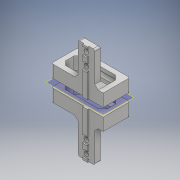
# Autodesk Inventor part: Estrutura - Suporte Mesa
Saved by Autodesk Inventor 2017 (Build 210142000, 142)
## iProperties
Created: 2020-08-23
Part Number: Estrutura - Suporte Mesa
Material: Generic
Document SubType Name: Modeling
Designer: ale
Density: 1 g/cm^3
Appearance: Default
Author: ale
Autodesk Inventor part; units mm, degrees
ref_plane "YZ Plane" through (0, 0, 0) normal (1, 0, 0) x (0, 1, 0)
ref_plane "XZ Plane" through (0, 0, 0) normal (0, 1, 0) x (-1, 0, 0)
ref_plane "XY Plane" through (0, 0, 0) normal (0, 0, 1) x (1, 0, 0)
sketch "Sketch1" plane through (0, 0, 0) normal (0, 0, 1) x (1, 0, 0)
  line L0 (-12.2491, 0) -> (12.2491, 0)
  line L1 (0, 10.917) -> (0, -10.917)
  line L2 (-40, -10) -> (-40, -16)
  line L3 (-40, -16) -> (16, -16)
  line L4 (-40, -10) -> (10, -10)
  line L5 (10, -10) -> (10, 10)
  line L6 (10, 10) -> (-40, 10)
  line L7 (-40, 10) -> (-40, 16)
  line L8 (-40, 16) -> (16, 16)
  line L9 (16, 16) -> (16, -16)
  point P0 (0, 0)
  point P1 (0, 0)
  dimension "d0" = 10
  dimension "d1" = 10
  dimension "d2" = 10
  dimension "d3" = 40
  dimension "d4" = 6
  dimension "d5" = 6
  dimension "d6" = 50
  dimension "d7" = 6
  constraints: 20 end point, 6 perpendicular, 2 horizontal, 2 midpoint, 2 vertical, 1 coincident
  measures "d0" distance between parallel lines of L6 L0
  measures "d1" distance between parallel lines of L4 L0
  measures "d2" distance between parallel lines of L5 L1
  measures "d3" distance between parallel lines of L2 L1
  measures "d4" distance between parallel lines of L3 L4
  measures "d5" distance between parallel lines of L9 L5
  measures "d6" distance between parallel lines of L7 L5
  measures "d7" distance between parallel lines of L6 L8
extrude "Extrusion1" add sketch "Sketch1" along normal blind 15 contours L5 L6 L7 L8 L9 L3 L2 L4
sketch "Sketch4" plane through (-40, 16, 0) normal (0, 1, 0) x (1, 0, 0)
  arc A0 (6, -4.25) -> (6, -10.75) centre (6, -7.5) ccw
  line L0 (0, 0) -> (0, -15) projected
  line L1 (56, 0) -> (0, 0) projected
  arc A1 (46, -10.75) -> (46, -4.25) centre (46, -7.5) ccw
  line L2 (56, -15) -> (0, -15) projected
  line L3 (46, -4.25) -> (6, -4.25)
  line L4 (46, -10.75) -> (6, -10.75)
  point P0 (40, 0)
  dimension "d22" = 6.5
  dimension "d23" = 6
  dimension "d24" = 7.5
  dimension "d25" = 6.5
  dimension "d26" = 46
  dimension "d27" = 7.5
  constraints: 4 end point, 4 point on circle, 4 tangent, 2 centre point
  measures "d22" diameter of A0
  measures "d23" distance from line of L0 A0.centre
  measures "d24" distance from line of L1 A0.centre
  measures "d25" diameter of A1
  measures "d26" distance from line of L0 A1.centre
  measures "d27" distance from line of L2 A1.centre
extrude "Extrusion3" cut sketch "Sketch4" against normal up to surface (6 mm away)
sketch "Sketch5" plane through (-40, -16, 0) normal (-1, 0, 0) x (0, 0, 1)
  line L0 (0, 0) -> (0, 32) projected
  line L1 (15, 6) -> (15, 0) projected
  line L2 (0, 32) -> (15, 32)
  line L3 (15, 32) -> (15, 0)
  line L4 (15, 0) -> (0, 0)
  line L5 (0, 0) -> (0, 32)
  point P0 (0, 16)
  constraints: 8 end point, 2 parallel, 1 horizontal, 1 perpendicular
extrude "Extrusion4" add sketch "Sketch5" along normal blind 6
sketch "Sketch6" plane through (16, -16, 0) normal (0, -1, 0) x (1, 0, 0)
  line L0 (-10, 0) -> (-30, 0)
  line L1 (-30, 0) -> (-30, 55)
  line L2 (-30, 55) -> (-10, 55)
  line L3 (-10, 55) -> (-10, 0)
  line L4 (-62, 0) -> (-62, 15) projected
  line L5 (0, 15) -> (-62, 15) projected
  point P0 (-16, 0)
  dimension "d43" = 20
  dimension "d44" = 55
  dimension "d76" = 52
  dimension "d77" = 15
  constraints: 8 end point, 2 parallel, 1 horizontal, 1 perpendicular
  measures "d43" distance of L1.end L2.end
  measures "d44" distance of L0.end L1.end
  measures "d76" distance between parallel lines of L3 L4
  measures "d77" distance between parallel lines of L0 L5
extrude "Extrusion5" add sketch "Sketch6" against normal blind 6
sketch "Sketch7" plane through (-46, -16, 0) normal (0, -1, 0) x (1, 0, 0)
  line L0 (32, 55) -> (52, 55) projected
  line L1 (56, 0) -> (6, 0) projected
  line L2 (39, 55) -> (39, 0)
  line L3 (45, 55) -> (45, 0)
  line L4 (39, 55) -> (45, 55)
  line L5 (45, 0) -> (39, 0)
  line L6 (0, 0) -> (0, 15) projected
  point P0 (46, 0)
  dimension "d78" = 45
  dimension "d79" = 6
  constraints: 8 end point, 2 collinear
  measures "d78" distance between parallel lines of L6 L3
  measures "d79" distance between parallel lines of L2 L3
extrude "Extrusion6" add sketch "Sketch7" along normal blind 1.5
sketch "Sketch8" plane through (-46, -17.5, 0) normal (0, -1, 0) x (1, 0, 0)
  line L0 (62, 0) -> (62, 15) projected
  line L1 (45, 55) -> (39, 55) projected
  point P0 (46, 0)
  point P1 (42, 48)
  point P2 (52, 55)
  point P3 (42, 33)
  dimension "d55" = 20
  dimension "d56" = 7
  dimension "d66" = 22
  dimension "d67" = 20
  constraints: 1 other
  measures "d56" distance from line of L1 point (42, 48)
  measures "d66" distance from line of point (42, 33) L1
hole "Hole2" at (-4, -17.5, 48) at (-4, -17.5, 33) direction (0, 1, 0) diameter 5.5 end through all counterbore diameter 10 counterbore depth 1.5
chamfer "Chamfer3" distance 5 angle 45 4 edges at (-40, -10, 7.5) (-40, 10, 7.5) (10, 10, 7.5) (10, -10, 7.5)
fillet "Fillet4" radius 2 5 edges at (-46, 16, 7.5) (16, 16, 7.5) (-46, -16, 7.5) (6, -12.5, 55) (-14, -13, 55)
chamfer "Chamfer4" distance 4 angle 45 2 edges at (6, -12.5, 15) (-14, -13, 15)
ref_plane "Work Plane2" through (0, 0, -5) normal (0, 0, -1) x (-1, 0, 0)
mirror "Mirror2" about plane through (0, 0, -5) normal (0, 0, -1)
body "Solid1"
